Autodesk Inventor part; units mm, degrees
(part 2 of 2)
  line L927 (205.0254, 75.1492) -> (204.2254, 75.1492)
  line L928 (204.2254, 75.1492) -> (204.2254, 72.0497)
  line L929 (204.2254, 72.0497) -> (205.0254, 72.0497)
  line L930 (205.0254, 72.0497) -> (205.0254, 66.2496)
  line L931 (205.0254, 66.2496) -> (204.2254, 66.2496)
  line L932 (204.2254, 66.2496) -> (204.2254, 63.1491)
  line L933 (204.2254, 63.1491) -> (205.0254, 63.1491)
  line L934 (205.0254, 63.1491) -> (205.0254, 62.15)
  line L935 (205.0254, 62.15) -> (219.0244, 62.15)
  line L936 (219.0244, 62.15) -> (219.0244, 63.1491)
  line L937 (219.0244, 63.1491) -> (219.8254, 63.1491)
  line L938 (219.8254, 63.1491) -> (219.8254, 66.2496)
  line L939 (219.8254, 66.2496) -> (219.0244, 66.2496)
  line L940 (219.0244, 66.2496) -> (219.0244, 72.0497)
  line L941 (219.0244, 72.0497) -> (219.8254, 72.0497)
  line L942 (219.8254, 72.0497) -> (219.8254, 75.1492)
  line L943 (219.8254, 75.1492) -> (219.0244, 75.1492)
  line L944 (219.0244, 75.1492) -> (219.0244, 76.1493)
  line L945 (219.0244, 76.1493) -> (205.0254, 76.1493)
  line L946 (224.0754, 76.1493) -> (224.0754, 75.1492)
  line L947 (224.0754, 75.1492) -> (223.2754, 75.1492)
  line L948 (223.2754, 75.1492) -> (223.2754, 72.0497)
  line L949 (223.2754, 72.0497) -> (224.0754, 72.0497)
  line L950 (224.0754, 72.0497) -> (224.0754, 66.2496)
  line L951 (224.0754, 66.2496) -> (223.2754, 66.2496)
  line L952 (223.2754, 66.2496) -> (223.2754, 63.1491)
  line L953 (223.2754, 63.1491) -> (224.0754, 63.1491)
  line L954 (224.0754, 63.1491) -> (224.0754, 62.15)
  line L955 (224.0754, 62.15) -> (238.0744, 62.15)
  line L956 (238.0744, 62.15) -> (238.0744, 63.1491)
  line L957 (238.0744, 63.1491) -> (238.8754, 63.1491)
  line L958 (238.8754, 63.1491) -> (238.8754, 66.2496)
  line L959 (238.8754, 66.2496) -> (238.0744, 66.2496)
  line L960 (238.0744, 66.2496) -> (238.0744, 72.0497)
  line L961 (238.0744, 72.0497) -> (238.8754, 72.0497)
  line L962 (238.8754, 72.0497) -> (238.8754, 75.1492)
  line L963 (238.8754, 75.1492) -> (238.0744, 75.1492)
  line L964 (238.0744, 75.1492) -> (238.0744, 76.1493)
  line L965 (238.0744, 76.1493) -> (224.0754, 76.1493)
  line L966 (243.1254, 76.1493) -> (243.1254, 75.1492)
  line L967 (243.1254, 75.1492) -> (242.3254, 75.1492)
  line L968 (242.3254, 75.1492) -> (242.3254, 72.0497)
  line L969 (242.3254, 72.0497) -> (243.1254, 72.0497)
  line L970 (243.1254, 72.0497) -> (243.1254, 66.2496)
  line L971 (243.1254, 66.2496) -> (242.3254, 66.2496)
  line L972 (242.3254, 66.2496) -> (242.3254, 63.1491)
  line L973 (242.3254, 63.1491) -> (243.1254, 63.1491)
  line L974 (243.1254, 63.1491) -> (243.1254, 62.15)
  line L975 (243.1254, 62.15) -> (257.1244, 62.15)
  line L976 (257.1244, 62.15) -> (257.1244, 63.1491)
  line L977 (257.1244, 63.1491) -> (257.9254, 63.1491)
  line L978 (257.9254, 63.1491) -> (257.9254, 66.2496)
  line L979 (257.9254, 66.2496) -> (257.1244, 66.2496)
  line L980 (257.1244, 66.2496) -> (257.1244, 72.0497)
  line L981 (257.1244, 72.0497) -> (257.9254, 72.0497)
  line L982 (257.9254, 72.0497) -> (257.9254, 75.1492)
  line L983 (257.9254, 75.1492) -> (257.1244, 75.1492)
  line L984 (257.1244, 75.1492) -> (257.1244, 76.1493)
  line L985 (257.1244, 76.1493) -> (243.1254, 76.1493)
  line L986 (266.9374, 76.1493) -> (266.9374, 75.1492)
  line L987 (266.9374, 75.1492) -> (266.1364, 75.1492)
  line L988 (266.1364, 75.1492) -> (266.1364, 72.0497)
  line L989 (266.1364, 72.0497) -> (266.9374, 72.0497)
  line L990 (266.9374, 72.0497) -> (266.9374, 66.2496)
  line L991 (266.9374, 66.2496) -> (266.1364, 66.2496)
  line L992 (266.1364, 66.2496) -> (266.1364, 63.1491)
  line L993 (266.1364, 63.1491) -> (266.9374, 63.1491)
  line L994 (266.9374, 63.1491) -> (266.9374, 62.15)
  line L995 (266.9374, 62.15) -> (280.9374, 62.15)
  line L996 (280.9374, 62.15) -> (280.9374, 63.1491)
  line L997 (280.9374, 63.1491) -> (281.7374, 63.1491)
  line L998 (281.7374, 63.1491) -> (281.7374, 66.2496)
  line L999 (281.7374, 66.2496) -> (280.9374, 66.2496)
  line L1000 (280.9374, 66.2496) -> (280.9374, 72.0497)
  line L1001 (280.9374, 72.0497) -> (281.7374, 72.0497)
  line L1002 (281.7374, 72.0497) -> (281.7374, 75.1492)
  line L1003 (281.7374, 75.1492) -> (280.9374, 75.1492)
  line L1004 (280.9374, 75.1492) -> (280.9374, 76.1493)
  line L1005 (280.9374, 76.1493) -> (266.9374, 76.1493)
  line L1006 (262.1754, 95.1993) -> (262.1754, 94.1992)
  line L1007 (262.1754, 94.1992) -> (261.3754, 94.1992)
  line L1008 (261.3754, 94.1992) -> (261.3754, 93.7293)
  line L1009 (261.3754, 93.7293) -> (253.9004, 93.7293)
  line L1010 (253.9004, 93.7293) -> (253.9004, 90.4989)
  line L1011 (253.9004, 90.4989) -> (253.0744, 90.4989)
  line L1012 (253.0744, 90.4989) -> (253.0744, 87.6989)
  line L1013 (253.0744, 87.6989) -> (253.9004, 87.6989)
  line L1014 (253.9004, 87.6989) -> (253.9004, 81.4286)
  line L1015 (253.9004, 81.4286) -> (255.6234, 81.4286)
  line L1016 (255.6234, 81.4286) -> (255.6234, 80.2299)
  line L1017 (255.6234, 80.2299) -> (258.9254, 80.2299)
  line L1018 (258.9254, 80.2299) -> (258.9254, 81.4286)
  line L1019 (258.9254, 81.4286) -> (260.6494, 81.4286)
  line L1020 (260.6494, 81.4286) -> (260.6494, 82.1991)
  line L1021 (260.6494, 82.1991) -> (262.1754, 82.1991)
  line L1022 (262.1754, 82.1991) -> (262.1754, 81.2)
  line L1023 (262.1754, 81.2) -> (276.1744, 81.2)
  line L1024 (276.1744, 81.2) -> (276.1744, 82.1991)
  line L1025 (276.1744, 82.1991) -> (277.7004, 82.1991)
  line L1026 (277.7004, 82.1991) -> (277.7004, 81.4286)
  line L1027 (277.7004, 81.4286) -> (279.4254, 81.4286)
  line L1028 (279.4254, 81.4286) -> (279.4254, 80.2299)
  line L1029 (279.4254, 80.2299) -> (282.7254, 80.2299)
  line L1030 (282.7254, 80.2299) -> (282.7254, 81.4286)
  line L1031 (282.7254, 81.4286) -> (284.4494, 81.4286)
  line L1032 (284.4494, 81.4286) -> (284.4494, 87.6989)
  line L1033 (284.4494, 87.6989) -> (285.2754, 87.6989)
  line L1034 (285.2754, 87.6989) -> (285.2754, 90.4989)
  line L1035 (285.2754, 90.4989) -> (284.4494, 90.4989)
  line L1036 (284.4494, 90.4989) -> (284.4494, 93.7293)
  line L1037 (284.4494, 93.7293) -> (276.9754, 93.7293)
  line L1038 (276.9754, 93.7293) -> (276.9754, 94.1992)
  line L1039 (276.9754, 94.1992) -> (276.1744, 94.1992)
  line L1040 (276.1744, 94.1992) -> (276.1744, 95.1993)
  line L1041 (276.1744, 95.1993) -> (262.1754, 95.1993)
  line L1042 (5, 95.1993) -> (5, 94.1992)
  line L1043 (5, 94.1992) -> (4.2007, 94.1992)
  line L1044 (4.2007, 94.1992) -> (4.2007, 91.0997)
  line L1045 (4.2007, 91.0997) -> (5, 91.0997)
  line L1046 (5, 91.0997) -> (5, 85.2996)
  line L1047 (0, 97.1993) -> (0, 3)
  line L1048 (5, 85.2996) -> (4.2007, 85.2996)
  line L1049 (4.2007, 85.2996) -> (4.2007, 82.1991)
  line L1050 (4.2007, 82.1991) -> (5, 82.1991)
  line L1051 (5, 82.1991) -> (5, 81.2)
  line L1052 (5, 81.2) -> (18.9996, 81.2)
  line L1053 (18.9996, 81.2) -> (18.9996, 82.1991)
  line L1054 (18.9996, 82.1991) -> (19.8002, 82.1991)
  line L1055 (19.8002, 82.1991) -> (19.8002, 85.2996)
  line L1056 (19.8002, 85.2996) -> (18.9996, 85.2996)
  line L1057 (18.9996, 85.2996) -> (18.9996, 91.0997)
  line L1058 (18.9996, 91.0997) -> (19.8002, 91.0997)
  line L1059 (19.8002, 91.0997) -> (19.8002, 94.1992)
  line L1060 (19.8002, 94.1992) -> (18.9996, 94.1992)
  line L1061 (18.9996, 94.1992) -> (18.9996, 95.1993)
  line L1062 (18.9996, 95.1993) -> (5, 95.1993)
  line L1063 (24.0501, 95.1993) -> (24.0501, 94.1992)
  line L1064 (24.0501, 94.1992) -> (23.2508, 94.1992)
  line L1065 (23.2508, 94.1992) -> (23.2508, 91.0997)
  line L1066 (23.2508, 91.0997) -> (24.0501, 91.0997)
  line L1067 (24.0501, 91.0997) -> (24.0501, 85.2996)
  line L1068 (24.0501, 85.2996) -> (23.2508, 85.2996)
  line L1069 (23.2508, 85.2996) -> (23.2508, 82.1991)
  line L1070 (23.2508, 82.1991) -> (24.0501, 82.1991)
  line L1071 (24.0501, 82.1991) -> (24.0501, 81.2)
  line L1072 (24.0501, 81.2) -> (38.0494, 81.2)
  line L1073 (38.0494, 81.2) -> (38.0494, 82.1991)
  line L1074 (38.0494, 82.1991) -> (38.8502, 82.1991)
  line L1075 (38.8502, 82.1991) -> (38.8502, 85.2996)
  line L1076 (38.8502, 85.2996) -> (38.0494, 85.2996)
  line L1077 (38.0494, 85.2996) -> (38.0494, 91.0997)
  line L1078 (38.0494, 91.0997) -> (38.8502, 91.0997)
  line L1079 (38.8502, 91.0997) -> (38.8502, 94.1992)
  line L1080 (38.8502, 94.1992) -> (38.0494, 94.1992)
  line L1081 (38.0494, 94.1992) -> (38.0494, 95.1993)
  line L1082 (38.0494, 95.1993) -> (24.0501, 95.1993)
  line L1083 (287.7004, 100.1993) -> (3, 100.1993)
  arc A3 (3, 100.1993) -> (0, 97.1993) centre (3, 97.1993) ccw
  line L1084 (43.1001, 95.1993) -> (43.1001, 94.1992)
  line L1085 (43.1001, 94.1992) -> (42.3007, 94.1992)
  line L1086 (42.3007, 94.1992) -> (42.3007, 91.0997)
  line L1087 (42.3007, 91.0997) -> (43.1001, 91.0997)
  line L1088 (43.1001, 91.0997) -> (43.1001, 85.2996)
  line L1089 (43.1001, 85.2996) -> (42.3007, 85.2996)
  line L1090 (42.3007, 85.2996) -> (42.3007, 82.1991)
  line L1091 (42.3007, 82.1991) -> (43.1001, 82.1991)
  line L1092 (43.1001, 82.1991) -> (43.1001, 81.2)
  line L1093 (43.1001, 81.2) -> (57.0994, 81.2)
  line L1094 (57.0994, 81.2) -> (57.0994, 82.1991)
  line L1095 (57.0994, 82.1991) -> (57.9002, 82.1991)
  line L1096 (57.9002, 82.1991) -> (57.9002, 85.2996)
  line L1097 (57.9002, 85.2996) -> (57.0994, 85.2996)
  line L1098 (57.0994, 85.2996) -> (57.0994, 91.0997)
  line L1099 (57.0994, 91.0997) -> (57.9002, 91.0997)
  line L1100 (57.9002, 91.0997) -> (57.9002, 94.1992)
  line L1101 (57.9002, 94.1992) -> (57.0994, 94.1992)
  line L1102 (57.0994, 94.1992) -> (57.0994, 95.1993)
  line L1103 (57.0994, 95.1993) -> (43.1001, 95.1993)
  line L1104 (62.1501, 95.1993) -> (62.1501, 94.1992)
  line L1105 (62.1501, 94.1992) -> (61.3507, 94.1992)
  line L1106 (61.3507, 94.1992) -> (61.3507, 91.0997)
  line L1107 (61.3507, 91.0997) -> (62.1501, 91.0997)
  line L1108 (62.1501, 91.0997) -> (62.1501, 85.2996)
  line L1109 (62.1501, 85.2996) -> (61.3507, 85.2996)
  line L1110 (61.3507, 85.2996) -> (61.3507, 82.1991)
  line L1111 (61.3507, 82.1991) -> (62.1501, 82.1991)
  line L1112 (62.1501, 82.1991) -> (62.1501, 81.2)
  line L1113 (62.1501, 81.2) -> (76.1494, 81.2)
  line L1114 (76.1494, 81.2) -> (76.1494, 82.1991)
  line L1115 (76.1494, 82.1991) -> (76.9502, 82.1991)
  line L1116 (76.9502, 82.1991) -> (76.9502, 85.2996)
  line L1117 (76.9502, 85.2996) -> (76.1494, 85.2996)
  line L1118 (76.1494, 85.2996) -> (76.1494, 91.0997)
  line L1119 (76.1494, 91.0997) -> (76.9502, 91.0997)
  line L1120 (76.9502, 91.0997) -> (76.9502, 94.1992)
  line L1121 (76.9502, 94.1992) -> (76.1494, 94.1992)
  line L1122 (76.1494, 94.1992) -> (76.1494, 95.1993)
  line L1123 (76.1494, 95.1993) -> (62.1501, 95.1993)
  line L1124 (81.2001, 95.1993) -> (81.2001, 94.1992)
  line L1125 (81.2001, 94.1992) -> (80.4007, 94.1992)
  line L1126 (80.4007, 94.1992) -> (80.4007, 91.0997)
  line L1127 (80.4007, 91.0997) -> (81.2001, 91.0997)
  line L1128 (81.2001, 91.0997) -> (81.2001, 85.2996)
  line L1129 (81.2001, 85.2996) -> (80.4007, 85.2996)
  line L1130 (80.4007, 85.2996) -> (80.4007, 82.1991)
  line L1131 (80.4007, 82.1991) -> (81.2001, 82.1991)
  line L1132 (81.2001, 82.1991) -> (81.2001, 81.2)
  line L1133 (81.2001, 81.2) -> (95.1994, 81.2)
  line L1134 (95.1994, 81.2) -> (95.1994, 82.1991)
  line L1135 (95.1994, 82.1991) -> (95.9988, 82.1991)
  line L1136 (95.9988, 82.1991) -> (95.9988, 85.2996)
  line L1137 (95.9988, 85.2996) -> (95.1994, 85.2996)
  line L1138 (95.1994, 85.2996) -> (95.1994, 91.0997)
  line L1139 (95.1994, 91.0997) -> (95.9988, 91.0997)
  line L1140 (95.9988, 91.0997) -> (95.9988, 94.1992)
  line L1141 (95.9988, 94.1992) -> (95.1994, 94.1992)
  line L1142 (95.1994, 94.1992) -> (95.1994, 95.1993)
  line L1143 (95.1994, 95.1993) -> (81.2001, 95.1993)
  line L1144 (100.2487, 95.1993) -> (100.2487, 94.1992)
  line L1145 (100.2487, 94.1992) -> (99.4507, 94.1992)
  line L1146 (99.4507, 94.1992) -> (99.4507, 91.0997)
  line L1147 (99.4507, 91.0997) -> (100.2487, 91.0997)
  line L1148 (100.2487, 91.0997) -> (100.2487, 85.2996)
  line L1149 (100.2487, 85.2996) -> (99.4507, 85.2996)
  line L1150 (99.4507, 85.2996) -> (99.4507, 82.1991)
  line L1151 (99.4507, 82.1991) -> (100.2487, 82.1991)
  line L1152 (100.2487, 82.1991) -> (100.2487, 81.2)
  line L1153 (100.2487, 81.2) -> (114.2494, 81.2)
  line L1154 (114.2494, 81.2) -> (114.2494, 82.1991)
  line L1155 (114.2494, 82.1991) -> (115.0484, 82.1991)
  line L1156 (115.0484, 82.1991) -> (115.0484, 85.2996)
  line L1157 (115.0484, 85.2996) -> (114.2494, 85.2996)
  line L1158 (114.2494, 85.2996) -> (114.2494, 91.0997)
  line L1159 (114.2494, 91.0997) -> (115.0484, 91.0997)
  line L1160 (115.0484, 91.0997) -> (115.0484, 94.1992)
  line L1161 (115.0484, 94.1992) -> (114.2494, 94.1992)
  line L1162 (114.2494, 94.1992) -> (114.2494, 95.1993)
  line L1163 (114.2494, 95.1993) -> (100.2487, 95.1993)
  line L1164 (119.2984, 95.1993) -> (119.2984, 94.1992)
  line L1165 (119.2984, 94.1992) -> (118.4994, 94.1992)
  line L1166 (118.4994, 94.1992) -> (118.4994, 91.0997)
  line L1167 (118.4994, 91.0997) -> (119.2984, 91.0997)
  line L1168 (119.2984, 91.0997) -> (119.2984, 85.2996)
  line L1169 (119.2984, 85.2996) -> (118.4994, 85.2996)
  line L1170 (118.4994, 85.2996) -> (118.4994, 82.1991)
  line L1171 (118.4994, 82.1991) -> (119.2984, 82.1991)
  line L1172 (119.2984, 82.1991) -> (119.2984, 81.2)
  line L1173 (119.2984, 81.2) -> (133.2994, 81.2)
  line L1174 (133.2994, 81.2) -> (133.2994, 82.1991)
  line L1175 (133.2994, 82.1991) -> (134.1004, 82.1991)
  line L1176 (134.1004, 82.1991) -> (134.1004, 85.2996)
  line L1177 (134.1004, 85.2996) -> (133.2994, 85.2996)
  line L1178 (133.2994, 85.2996) -> (133.2994, 91.0997)
  line L1179 (133.2994, 91.0997) -> (134.1004, 91.0997)
  line L1180 (134.1004, 91.0997) -> (134.1004, 94.1992)
  line L1181 (134.1004, 94.1992) -> (133.2994, 94.1992)
  line L1182 (133.2994, 94.1992) -> (133.2994, 95.1993)
  line L1183 (133.2994, 95.1993) -> (119.2984, 95.1993)
  line L1184 (138.3504, 95.1993) -> (138.3504, 94.1992)
  line L1185 (138.3504, 94.1992) -> (137.5504, 94.1992)
  line L1186 (137.5504, 94.1992) -> (137.5504, 91.0997)
  line L1187 (137.5504, 91.0997) -> (138.3504, 91.0997)
  line L1188 (138.3504, 91.0997) -> (138.3504, 85.2996)
  line L1189 (138.3504, 85.2996) -> (137.5504, 85.2996)
  line L1190 (137.5504, 85.2996) -> (137.5504, 82.1991)
  line L1191 (137.5504, 82.1991) -> (138.3504, 82.1991)
  line L1192 (138.3504, 82.1991) -> (138.3504, 81.2)
  line L1193 (138.3504, 81.2) -> (152.3494, 81.2)
  line L1194 (152.3494, 81.2) -> (152.3494, 82.1991)
  line L1195 (152.3494, 82.1991) -> (153.1504, 82.1991)
  line L1196 (153.1504, 82.1991) -> (153.1504, 85.2996)
  line L1197 (153.1504, 85.2996) -> (152.3494, 85.2996)
  line L1198 (152.3494, 85.2996) -> (152.3494, 91.0997)
  line L1199 (152.3494, 91.0997) -> (153.1504, 91.0997)
  line L1200 (153.1504, 91.0997) -> (153.1504, 94.1992)
  line L1201 (153.1504, 94.1992) -> (152.3494, 94.1992)
  line L1202 (152.3494, 94.1992) -> (152.3494, 95.1993)
  line L1203 (152.3494, 95.1993) -> (138.3504, 95.1993)
  line L1204 (157.4004, 95.1993) -> (157.4004, 94.1992)
  line L1205 (157.4004, 94.1992) -> (156.6004, 94.1992)
  line L1206 (156.6004, 94.1992) -> (156.6004, 91.0997)
  line L1207 (156.6004, 91.0997) -> (157.4004, 91.0997)
  line L1208 (157.4004, 91.0997) -> (157.4004, 85.2996)
  line L1209 (157.4004, 85.2996) -> (156.6004, 85.2996)
  line L1210 (156.6004, 85.2996) -> (156.6004, 82.1991)
  line L1211 (156.6004, 82.1991) -> (157.4004, 82.1991)
  line L1212 (157.4004, 82.1991) -> (157.4004, 81.2)
  line L1213 (157.4004, 81.2) -> (171.3994, 81.2)
  line L1214 (171.3994, 81.2) -> (171.3994, 82.1991)
  line L1215 (171.3994, 82.1991) -> (172.2004, 82.1991)
  line L1216 (172.2004, 82.1991) -> (172.2004, 85.2996)
  line L1217 (172.2004, 85.2996) -> (171.3994, 85.2996)
  line L1218 (171.3994, 85.2996) -> (171.3994, 91.0997)
  line L1219 (171.3994, 91.0997) -> (172.2004, 91.0997)
  line L1220 (172.2004, 91.0997) -> (172.2004, 94.1992)
  line L1221 (172.2004, 94.1992) -> (171.3994, 94.1992)
  line L1222 (171.3994, 94.1992) -> (171.3994, 95.1993)
  line L1223 (171.3994, 95.1993) -> (157.4004, 95.1993)
  line L1224 (176.4504, 95.1993) -> (176.4504, 94.1992)
  line L1225 (176.4504, 94.1992) -> (175.6504, 94.1992)
  line L1226 (175.6504, 94.1992) -> (175.6504, 91.0997)
  line L1227 (175.6504, 91.0997) -> (176.4504, 91.0997)
  line L1228 (176.4504, 91.0997) -> (176.4504, 85.2996)
  line L1229 (176.4504, 85.2996) -> (175.6504, 85.2996)
  line L1230 (175.6504, 85.2996) -> (175.6504, 82.1991)
  line L1231 (175.6504, 82.1991) -> (176.4504, 82.1991)
  line L1232 (176.4504, 82.1991) -> (176.4504, 81.2)
  line L1233 (176.4504, 81.2) -> (190.4494, 81.2)
  line L1234 (190.4494, 81.2) -> (190.4494, 82.1991)
  line L1235 (190.4494, 82.1991) -> (191.2504, 82.1991)
  line L1236 (191.2504, 82.1991) -> (191.2504, 85.2996)
  line L1237 (191.2504, 85.2996) -> (190.4494, 85.2996)
  line L1238 (190.4494, 85.2996) -> (190.4494, 91.0997)
  line L1239 (190.4494, 91.0997) -> (191.2504, 91.0997)
  line L1240 (191.2504, 91.0997) -> (191.2504, 94.1992)
  line L1241 (191.2504, 94.1992) -> (190.4494, 94.1992)
  line L1242 (190.4494, 94.1992) -> (190.4494, 95.1993)
  line L1243 (190.4494, 95.1993) -> (176.4504, 95.1993)
  line L1244 (195.5004, 95.1993) -> (195.5004, 94.1992)
  line L1245 (195.5004, 94.1992) -> (194.7004, 94.1992)
  line L1246 (194.7004, 94.1992) -> (194.7004, 91.0997)
  line L1247 (194.7004, 91.0997) -> (195.5004, 91.0997)
  line L1248 (195.5004, 91.0997) -> (195.5004, 85.2996)
  line L1249 (195.5004, 85.2996) -> (194.7004, 85.2996)
  line L1250 (194.7004, 85.2996) -> (194.7004, 82.1991)
  line L1251 (194.7004, 82.1991) -> (195.5004, 82.1991)
  line L1252 (195.5004, 82.1991) -> (195.5004, 81.2)
  line L1253 (195.5004, 81.2) -> (209.4994, 81.2)
  line L1254 (209.4994, 81.2) -> (209.4994, 82.1991)
  line L1255 (209.4994, 82.1991) -> (210.3004, 82.1991)
  line L1256 (210.3004, 82.1991) -> (210.3004, 85.2996)
  line L1257 (210.3004, 85.2996) -> (209.4994, 85.2996)
  line L1258 (209.4994, 85.2996) -> (209.4994, 91.0997)
  line L1259 (209.4994, 91.0997) -> (210.3004, 91.0997)
  line L1260 (210.3004, 91.0997) -> (210.3004, 94.1992)
  line L1261 (210.3004, 94.1992) -> (209.4994, 94.1992)
  line L1262 (209.4994, 94.1992) -> (209.4994, 95.1993)
  line L1263 (209.4994, 95.1993) -> (195.5004, 95.1993)
  line L1264 (214.5504, 95.1993) -> (214.5504, 94.1992)
  line L1265 (214.5504, 94.1992) -> (213.7504, 94.1992)
  line L1266 (213.7504, 94.1992) -> (213.7504, 91.0997)
  line L1267 (213.7504, 91.0997) -> (214.5504, 91.0997)
  line L1268 (214.5504, 91.0997) -> (214.5504, 85.2996)
  line L1269 (214.5504, 85.2996) -> (213.7504, 85.2996)
  line L1270 (213.7504, 85.2996) -> (213.7504, 82.1991)
  line L1271 (213.7504, 82.1991) -> (214.5504, 82.1991)
  line L1272 (214.5504, 82.1991) -> (214.5504, 81.2)
  line L1273 (214.5504, 81.2) -> (228.5494, 81.2)
  line L1274 (228.5494, 81.2) -> (228.5494, 82.1991)
  line L1275 (228.5494, 82.1991) -> (229.3504, 82.1991)
  line L1276 (229.3504, 82.1991) -> (229.3504, 85.2996)
  line L1277 (229.3504, 85.2996) -> (228.5494, 85.2996)
  line L1278 (228.5494, 85.2996) -> (228.5494, 91.0997)
  line L1279 (228.5494, 91.0997) -> (229.3504, 91.0997)
  line L1280 (229.3504, 91.0997) -> (229.3504, 94.1992)
  line L1281 (229.3504, 94.1992) -> (228.5494, 94.1992)
  line L1282 (228.5494, 94.1992) -> (228.5494, 95.1993)
  line L1283 (228.5494, 95.1993) -> (214.5504, 95.1993)
  line L1284 (233.6004, 95.1993) -> (233.6004, 94.1992)
  line L1285 (233.6004, 94.1992) -> (232.8004, 94.1992)
  line L1286 (232.8004, 94.1992) -> (232.8004, 91.0997)
  line L1287 (232.8004, 91.0997) -> (233.6004, 91.0997)
  line L1288 (233.6004, 91.0997) -> (233.6004, 85.2996)
  line L1289 (233.6004, 85.2996) -> (232.8004, 85.2996)
  line L1290 (232.8004, 85.2996) -> (232.8004, 82.1991)
  line L1291 (232.8004, 82.1991) -> (233.6004, 82.1991)
  line L1292 (233.6004, 82.1991) -> (233.6004, 81.2)
  line L1293 (233.6004, 81.2) -> (247.5994, 81.2)
  line L1294 (247.5994, 81.2) -> (247.5994, 82.1991)
  line L1295 (247.5994, 82.1991) -> (248.4004, 82.1991)
  line L1296 (248.4004, 82.1991) -> (248.4004, 85.2996)
  line L1297 (248.4004, 85.2996) -> (247.5994, 85.2996)
  line L1298 (247.5994, 85.2996) -> (247.5994, 91.0997)
  line L1299 (247.5994, 91.0997) -> (248.4004, 91.0997)
  line L1300 (248.4004, 91.0997) -> (248.4004, 94.1992)
  line L1301 (248.4004, 94.1992) -> (247.5994, 94.1992)
  line L1302 (247.5994, 94.1992) -> (247.5994, 95.1993)
  line L1303 (247.5994, 95.1993) -> (233.6004, 95.1993)
  circle A4 centre (287.7004, 97.1993) radius 1.5
  circle A5 centre (3, 97.1993) radius 1.5
  circle A6 centre (3, 3) radius 1.5
  circle A7 centre (287.7004, 3) radius 1.5
  line L1304 (26.7621, 60.0993) -> (26.7621, 78.2)
  line L1305 (30.5751, 78.2) -> (30.5751, 60.0993)
  line L1306 (29.1433, 41.0493) -> (29.1433, 60.0993)
  line L1307 (35.3376, 60.0993) -> (35.3376, 41.0493)
  line L1308 (260.1244, 60.0993) -> (260.1244, 78.2)
  line L1309 (263.9374, 78.2) -> (263.9374, 60.0993)
  line L1310 (236.3124, 21.9995) -> (236.3124, 40.1)
  line L1311 (243.7564, 40.1) -> (243.7564, 21.9995)
  line L1312 (89.8185, 21.05) -> (123.4424, 21.05)
  line L1313 (123.4424, 17.299) -> (89.8185, 17.299)
  line L1314 (177.0694, 17.299) -> (143.4434, 17.299)
  line L1315 (143.4434, 21.05) -> (177.0694, 21.05)
  line L1316 (194.8814, 21.05) -> (194.8814, 3)
  line L1317 (189.8184, 3) -> (189.8184, 21.05)
  line L1318 (218.6934, 21.05) -> (218.6934, 3)
  line L1319 (214.8804, 3) -> (214.8804, 21.05)
  line L1320 (242.5064, 21.9995) -> (242.5064, 3)
  line L1321 (238.6934, 3) -> (238.6934, 21.9995)
  line L1322 (266.3184, 21.05) -> (266.3184, 3)
  line L1323 (262.5054, 3) -> (262.5054, 21.05)
  line L1324 (44.8626, 40.1) -> (44.8626, 21.9995)
  line L1325 (42.1808, 21.9995) -> (42.1808, 40.1)
  line L1326 (9.1438, 59.15) -> (9.1438, 39.5791)
  line L1327 (3, 78.2) -> (3, 6)
  line L1328 (6.7625, 78.2) -> (6.7625, 59.15)
  line L1329 (77.0688, 21.05) -> (77.0688, 3)
  line L1330 (72.0057, 3) -> (72.0057, 21.05)
  line L1331 (52.0064, 21.05) -> (52.0064, 3)
  line L1332 (48.1932, 3) -> (48.1932, 21.05)
  line L1333 (28.1938, 21.05) -> (28.1938, 3)
  line L1334 (24.3808, 3) -> (24.3808, 21.05)
  line L1335 (4.3813, 21.9995) -> (4.3813, 6)
  line L1336 (5.6312, 39.5791) -> (5.6312, 21.9995)
  line L1337 (3, 78.2) -> (6.7625, 78.2)
  line L1338 (6.7625, 59.15) -> (9.1438, 59.15)
  line L1339 (9.1438, 39.5791) -> (5.6312, 39.5791)
  line L1340 (4.3813, 21.9995) -> (5.6312, 21.9995)
  line L1341 (3, 6) -> (4.3813, 6)
  line L1342 (35.3376, 41.0493) -> (29.1433, 41.0493)
  line L1343 (26.7621, 60.0993) -> (29.1433, 60.0993)
  line L1344 (30.5751, 60.0993) -> (35.3376, 60.0993)
  line L1345 (26.7621, 78.2) -> (30.5751, 78.2)
  line L1346 (42.1808, 40.1) -> (44.8626, 40.1)
  line L1347 (44.8626, 21.9995) -> (42.1808, 21.9995)
  line L1348 (283.9374, 58.6293) -> (283.9374, 78.4286)
  line L1349 (287.7004, 78.4286) -> (287.7004, 6)
  line L1350 (285.0684, 39.5791) -> (285.0684, 58.6293)
  line L1351 (280.3054, 21.9995) -> (280.3054, 39.5791)
  line L1352 (286.3184, 6) -> (286.3184, 21.9995)
  line L1353 (24.3808, 21.05) -> (28.1938, 21.05)
  line L1354 (48.1932, 21.05) -> (52.0064, 21.05)
  line L1355 (72.0057, 21.05) -> (77.0688, 21.05)
  line L1356 (89.8185, 17.299) -> (89.8185, 21.05)
  line L1357 (123.4424, 21.05) -> (123.4424, 17.299)
  line L1358 (89.8185, 6.7005) -> (123.4424, 6.7005)
  line L1359 (89.8185, 3) -> (89.8185, 6.7005)
  line L1360 (123.4424, 6.7005) -> (123.4424, 3)
  line L1361 (143.4434, 17.299) -> (143.4434, 21.05)
  line L1362 (177.0694, 21.05) -> (177.0694, 17.299)
  line L1363 (143.4434, 3) -> (143.4434, 6.7005)
  line L1364 (177.0694, 6.7005) -> (177.0694, 3)
  line L1365 (143.4434, 6.7005) -> (177.0694, 6.7005)
  line L1366 (189.8184, 21.05) -> (194.8814, 21.05)
  line L1367 (214.8804, 21.05) -> (218.6934, 21.05)
  line L1368 (238.6934, 21.9995) -> (236.3124, 21.9995)
  line L1369 (243.7564, 21.9995) -> (242.5064, 21.9995)
  line L1370 (245.8374, 39.5791) -> (245.8374, 59.15)
  line L1371 (248.5184, 59.15) -> (248.5184, 39.5791)
  line L1372 (236.3124, 40.1) -> (243.7564, 40.1)
  line L1373 (248.5184, 39.5791) -> (245.8374, 39.5791)
  line L1374 (245.8374, 59.15) -> (248.5184, 59.15)
  line L1375 (24.3808, 3) -> (28.1938, 3)
  line L1376 (48.1932, 3) -> (52.0064, 3)
  line L1377 (72.0057, 3) -> (77.0688, 3)
  line L1378 (89.8185, 3) -> (123.4424, 3)
  line L1379 (143.4434, 3) -> (177.0694, 3)
  line L1380 (189.8184, 3) -> (194.8814, 3)
  line L1381 (214.8804, 3) -> (218.6934, 3)
  line L1382 (238.6934, 3) -> (242.5064, 3)
  line L1383 (262.5054, 21.05) -> (266.3184, 21.05)
  line L1384 (287.7004, 6) -> (286.3184, 6)
  line L1385 (262.5054, 3) -> (266.3184, 3)
  line L1386 (286.3184, 21.9995) -> (280.3054, 21.9995)
  line L1387 (285.0684, 39.5791) -> (280.3054, 39.5791)
  line L1388 (285.0684, 58.6293) -> (283.9374, 58.6293)
  line L1389 (283.9374, 78.4286) -> (287.7004, 78.4286)
  line L1390 (260.1244, 78.2) -> (263.9374, 78.2)
  line L1391 (263.9374, 60.0993) -> (260.1244, 60.0993)
  line L1392 (254.2304, 37.049) -> (254.2304, 36.5791)
  line L1393 (269.8314, 37.049) -> (269.8314, 36.5791)
  line L1394 (253.5064, 25.049) -> (253.5064, 24.2787)
  line L1395 (270.5564, 25.049) -> (270.5564, 24.2787)
  line L1396 (16.1057, 37.049) -> (16.1057, 36.5791)
  line L1397 (31.7064, 37.049) -> (31.7064, 36.5791)
  line L1398 (32.4313, 25.049) -> (32.4313, 24.2787)
  line L1399 (15.3808, 25.049) -> (15.3808, 24.2787)
  point P0 (0, 0)
  constraints: 2800 end point, 8 centre point, 8 point on circle
extrude "Extrusion1" add sketch "Sketch1" along normal blind 3
body "Solid1"
